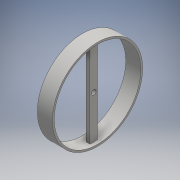
# Autodesk Inventor part: Molde2
Saved by Autodesk Inventor 2016 (Build 200138000, 138)
## iProperties
Created: 2019-03-18
Part Number: Molde2
Material: Genérico
Document SubType Name: Modeling
Designer: FIMCP
Density: 1 g/cm^3
Appearance: Valor por defecto
Author: FIMCP
Autodesk Inventor part; units mm, degrees
ref_plane "YZ Plane" through (0, 0, 0) normal (1, 0, 0) x (0, 1, 0)
ref_plane "XZ Plane" through (0, 0, 0) normal (0, 1, 0) x (-1, 0, 0)
ref_plane "XY Plane" through (0, 0, 0) normal (0, 0, 1) x (1, 0, 0)
sketch "Boceto1" plane through (0, 0, 0) normal (1, 0, 0) x (0, 1, 0)
  line L0 (2, 23) -> (-2, 23)
  line L1 (-2, 23) -> (-2, -23)
  line L2 (-2, -23) -> (2, -23)
  line L3 (2, -23) -> (2, 23)
  circle A0 centre (0, 0) radius 1.25
  dimension "d0" = 4
  dimension "d1" = 46
  dimension "d2" = 2
  dimension "d3" = 23
  dimension "d4" = 2.5
  constraints: 8 end point, 2 parallel, 1 centre point, 1 coincident, 1 horizontal, 1 perpendicular
  measures "d0" distance of L2.end L1.end
  measures "d1" distance of L1.end L0.end
  measures "d2" distance from line of point (0, 0) L3
  measures "d3" distance from line of point (0, 0) L2
  measures "d4" diameter of A0
extrude "Extrusión1" add sketch "Boceto1" along normal blind 2
sketch "Boceto2" plane through (0, 0, 0) normal (1, 0, 0) x (0, 1, 0)
  circle A0 centre (0, 0) radius 24
  circle A1 centre (0, 0) radius 23
  dimension "d7" = 48
  dimension "d8" = 46
  constraints: 2 centre point, 2 coincident
  measures "d7" diameter of A0
  measures "d8" diameter of A1
extrude "Extrusión2" add sketch "Boceto2" along normal mid plane 8
